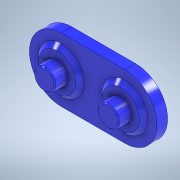
# Autodesk Inventor part: base
Saved by Autodesk Inventor 2022 (Build 260153000, 153)
## iProperties
Created: 2023-03-13
Part Number: base
Material: Genérico
Document SubType Name: Modeling
Designer: jpjoa
Density: 1 g/cm^3
Appearance: Azul - Tinta de parede - Com brilho
Author: jpjoa
Autodesk Inventor part; units mm, degrees
ref_plane "YZ Plane" through (0, 0, 0) normal (1, 0, 0) x (0, 1, 0)
ref_plane "XZ Plane" through (0, 0, 0) normal (0, 1, 0) x (-1, 0, 0)
ref_plane "XY Plane" through (0, 0, 0) normal (0, 0, 1) x (1, 0, 0)
sketch "Esboço1" plane through (0, 0, 0) normal (0, 0, 1) x (1, 0, 0)
  line L0 (0, 0) -> (60, 0) construction
  line L1 (0, 30) -> (60, 30)
  line L2 (60, -30) -> (0, -30)
  arc A0 (0, 30) -> (0, -30) centre (0, 0) ccw
  arc A1 (60, -30) -> (60, 30) centre (60, 0) ccw
  circle A2 centre (0, 0) radius 17.5
  circle A3 centre (0, 0) radius 10
  circle A4 centre (60, 0) radius 17.5
  circle A5 centre (60, 0) radius 10
  point P0 (30, 0)
  dimension "d0" = 60
  dimension "d1" = 60
  dimension "d2" = 30
  dimension "d3" = 35
  dimension "d4" = 20
  dimension "d11" = 35
  dimension "d12" = 20
  constraints: 8 end point, 6 centre point, 4 coincident, 4 point on circle, 4 tangent, 1 horizontal, 1 midpoint, 1 parallel
  measures "d0" distance of L0.start L0.end
  measures "d1" distance between parallel lines of L2 L1
  measures "d2" radius of A0
  measures "d3" diameter of A2
  measures "d4" diameter of A3
  measures "d11" diameter of A4
  measures "d12" diameter of A5
extrude "Extrusão1" add sketch "Esboço1" along normal blind 10 contours L1 A1 L2 A0 | A4 | A5
extrude "Extrusão2" add sketch "Esboço1" along normal blind 14 contours A2 | A4 | A5
extrude "Extrusão3" add sketch "Esboço1" along normal blind 26 contours A3 | A5
chamfer "Chanfro1" distance 4 angle 45 2 edges at (-17.5, 0, 10) (42.5, 0, 10)
chamfer "Chanfro2" distance 1 angle 45 2 edges at (-10, 0, 26) (50, 0, 26)
equation "\"d11\" = d3"
equation "\"d12\" = d4"
